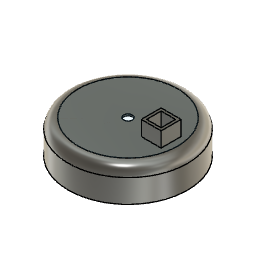
dumb_doorbell (Autodesk Fusion 360 design; units mm, degrees)
Autodesk Fusion 360 part; units mm, degrees
sketch "Sketch1" plane through (0, 0, 0) normal (0, 0, 1) x (1, 0, 0)
  circle A0 centre (0, 0) radius 2.65
  circle A1 centre (0, 0) radius 30
  dimension "d1" = 5.3
  dimension "d2" = 60
  constraint coincident A0.centre A1.centre
  constraint concentric A0 A1
  measures "d1" diameter of A0
  measures "d2" diameter of A1
extrude "Extrude1" add sketch "Sketch1" along normal blind 4
sketch "Sketch2" plane through (0, 0, 4) normal (0, 0, 1) x (-1, 0, 0)
  circle A0 centre (0, 0) radius 2.65
  circle A1 centre (0, 0) radius 30
sketch "Sketch3" plane through (0, 0, 4) normal (0, 0, 1) x (-1, 0, 0)
  line L0 (0, 0) -> (-20, 0)
  circle A0 centre (-20, 0) radius 2.05
  dimension "d5" = 20
  dimension "d6" = 4.1
  constraint coincident L0.start origin
  constraint horizontal L0
  constraint coincident L0.end A0.centre
  measures "d5" distance of L0.start L0.end
  measures "d6" diameter of A0
extrude "Extrude2" cut sketch "Sketch3" against normal blind 10
sketch "Sketch4" plane through (0, 0, 4) normal (0, 0, 1) x (-1, 0, 0)
  line L0 (-20, 0) -> (-20, 6)
  line L1 (-20, 6) -> (-26, 6)
  line L2 (-26, 6) -> (-26, -6)
  line L3 (-26, -6) -> (-20, -6)
  line L4 (-20, -6) -> (-20, 6)
  line L5 (-20, 6) -> (-14, 6)
  line L6 (-14, 6) -> (-14, -6)
  line L7 (-14, -6) -> (-20, -6)
  line L8 (-20, -6) -> (-20, 6)
  line L9 (-15.625, -4.375) -> (-24.375, -4.375)
  line L10 (-24.375, -4.375) -> (-24.375, 4.375)
  line L11 (-24.375, 4.375) -> (-15.625, 4.375)
  line L12 (-15.625, 4.375) -> (-15.625, -4.375)
  dimension "d9" = 6
  dimension "d10" = 6
  dimension "d11" = 12
  dimension "d12" = 6
  dimension "d13" = 12
  dimension "d14" = 1.625
  dimension "d15" = 1.625
  dimension "d16" = 1.625
  dimension "d17" = 1.625
  constraint vertical L0
  constraint horizontal L1
  constraint vertical L2
  constraint horizontal L3
  constraint vertical L4
  constraint horizontal L5
  constraint vertical L6
  constraint horizontal L7
  constraint vertical L8
  constraint horizontal L9
  constraint vertical L10
  constraint horizontal L11
  constraint vertical L12
  measures "d9" distance of L0.start L0.end
  measures "d10" distance of L2.end L3.end
  measures "d11" distance of L1.end L2.end
  measures "d12" distance of L0.end L5.end
  measures "d13" distance of L5.end L6.end
  measures "d14" distance of L2 L10
  measures "d15" distance of L6 L12
  measures "d16" distance of L7 L9
  measures "d17" distance of L1 L11
extrude "Extrude3" add sketch "Sketch4" along normal blind 9 contours L0 L1 L2 L3 L4 L8 L9 L10 L11 | L0 L4 L5 L6 L7 L8 L9 L11 L12
move_face "OffsetFaces1" offset -3 1 faces at (13.0263, -9.0432, 0)
sketch "Sketch5" plane through (0, 0, 0) normal (0, 1, 0) x (1, 0, 0)
  line L0 (30, -3) -> (30, 2)
  arc A0 (30, -3) -> (35, 2) centre (30, 2) ccw
  arc A1 (30, -4) -> (36, 2) centre (30, 2) ccw
  line L1 (35, 2) -> (35, 16)
  line L2 (35, 16) -> (36, 16)
  line L3 (36, 16) -> (36, 2)
  line L4 (-30, -3) -> (30, -3)
  line L5 (30, -4) -> (30, -3)
  dimension "d21" = 5
  dimension "d22" = 14
  dimension "d23" = 1
  constraint vertical L0
  constraint coincident L0.end A0.centre
  constraint tangent A0 L1
  constraint vertical L1
  constraint perpendicular L1 L2
  constraint tangent A1 L3
  measures "d21" distance of L0.start L0.end
  measures "d22" distance of A1.end L2.end
  measures "d23" distance of A1.start L4
revolve "Revolve1" add sketch "Sketch5" angle 360 about axis through (0, 0, 1.75) along (0, 0, 1)
